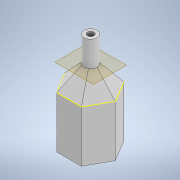
# Autodesk Inventor part: motorattacher
Saved by Autodesk Inventor 2022 (Build 260153000, 153)
## iProperties
Created: 2022-04-02
Part Number: motorattacher
Material: Generic
Document SubType Name: Modeling
Designer: moaze
Density: 1 g/cm^3
Appearance: Default
Author: moaze
Autodesk Inventor part; units mm, degrees
ref_plane "YZ Plane" through (0, 0, 0) normal (1, 0, 0) x (0, 1, 0)
ref_plane "XZ Plane" through (0, 0, 0) normal (0, 1, 0) x (-1, 0, 0)
ref_plane "XY Plane" through (0, 0, 0) normal (0, 0, 1) x (1, 0, 0)
sketch "Sketch1" plane through (0, 0, 0) normal (0, 1, 0) x (-1, 0, 0)
  line L0 (3.0315, -4.7903) -> (-2.5932, -4.7903)
  line L1 (-2.5932, -4.7903) -> (-5.3821, -0.0266)
  line L2 (-5.3821, -0.0266) -> (-2.721, 4.8097)
  line L3 (-2.721, 4.8097) -> (2.7981, 4.8097)
  line L4 (2.7981, 4.8097) -> (5.7396, 0.1397)
  line L5 (5.7396, 0.1397) -> (3.0315, -4.7903)
  line L6 (-7.5579, -0.0555) -> (-3.6782, -6.6826)
  line L7 (-3.6782, -6.6826) -> (4.1511, -6.6826)
  line L8 (4.1511, -6.6826) -> (7.9347, 0.2053)
  line L9 (7.9347, 0.2053) -> (3.8427, 6.7021)
  line L10 (3.8427, 6.7021) -> (-3.8397, 6.7021)
  line L11 (-3.8397, 6.7021) -> (-7.5579, -0.0555)
  line L12 (0.004, -1.2887) -> (0.004, -3.3542)
  dimension "d43" = 9.6
  constraints: 26 end point, 3 equal length, 2 perpendicular, 1 vertical, 5 other
  measures "d43" distance between parallel lines of L0 L3
ref_plane "Work Plane1" through (0, 14.35, 0) normal (0, 1, 0) x (1, 0, 0)
sketch "Sketch3" plane through (0, 14.35, 0) normal (0, 1, 0) x (1, 0, 0)
  circle A0 centre (0, 0) radius 2
  dimension "d7" = 4
  constraints: 1 centre point, 1 coincident
  measures "d7" diameter of A0
extrude "Extrusion3" add sketch "Sketch1" along normal blind 8
sketch "Sketch6" plane through (0, 8, 0) normal (0, 1, 0) x (1, 0, 0)
  line L0 (3.6782, 6.6826) -> (-4.1511, 6.6826) projected
  line L1 (-4.1511, 6.6826) -> (-7.9347, -0.2053) projected
  line L2 (-7.9347, -0.2053) -> (-3.8427, -6.7021) projected
  line L3 (-3.8427, -6.7021) -> (3.8397, -6.7021) projected
  line L4 (3.8397, -6.7021) -> (7.5579, 0.0555) projected
  line L5 (7.5579, 0.0555) -> (3.6782, 6.6826) projected
  line L6 (-3.0315, 4.7903) -> (2.5932, 4.7903) projected
  line L7 (2.5932, 4.7903) -> (5.3821, 0.0266) projected
  line L8 (5.3821, 0.0266) -> (2.721, -4.8097) projected
  line L9 (2.721, -4.8097) -> (-2.7981, -4.8097) projected
  line L10 (-2.7981, -4.8097) -> (-5.7396, -0.1397) projected
  line L11 (-5.7396, -0.1397) -> (-3.0315, 4.7903) projected
  point P0 (0, 0)
loft "Loft2" add profiles "Sketch3" section 1 edges at (-0.2365, 8, -6.6826) (-6.0429, 8, -3.2387) (-5.8887, 8, 3.4537) (-0.0015, 8, 6.7021) (5.6988, 8, 3.3233) (5.618, 8, -3.3691)
sketch "Sketch7" plane through (0, 14.35, 0) normal (0, 1, 0) x (0.9999645, 0, -0.0084267)
  arc A0 (1.0109, 1.7257) -> (-1.0109, 1.7257) centre (0, 0) ccw projected
  arc A1 (-1.0109, 1.7257) -> (-1.9997, -0.036) centre (0, 0) ccw projected
  arc A2 (-1.9997, -0.036) -> (-0.9777, -1.7447) centre (0, 0) ccw projected
  arc A3 (-0.9777, -1.7447) -> (1.0106, -1.7259) centre (0, 0) ccw projected
  arc A4 (1.0106, -1.7259) -> (2, -0.0025) centre (0, 0) ccw projected
  arc A5 (2, -0.0025) -> (1.0109, 1.7257) centre (0, 0) ccw projected
  point P0 (0, 0)
sketch "Sketch8" plane through (0, 0, 0) normal (0, -1, 0) x (1, 0, 0)
  line L0 (3.6782, -6.6826) -> (-4.1511, -6.6826) projected
  line L1 (7.5579, -0.0555) -> (3.6782, -6.6826) projected
  line L2 (3.8397, 6.7021) -> (7.5579, -0.0555) projected
  line L3 (-3.8427, 6.7021) -> (3.8397, 6.7021) projected
  line L4 (-7.9347, 0.2053) -> (-3.8427, 6.7021) projected
  line L5 (-4.1511, -6.6826) -> (-7.9347, 0.2053) projected
  line L6 (-3.0315, -4.7903) -> (2.5932, -4.7903) projected
  line L7 (-5.7396, 0.1397) -> (-3.0315, -4.7903) projected
  line L8 (-2.7981, 4.8097) -> (-5.7396, 0.1397) projected
  line L9 (2.721, 4.8097) -> (-2.7981, 4.8097) projected
  line L10 (5.3821, -0.0266) -> (2.721, 4.8097) projected
  line L11 (2.5932, -4.7903) -> (5.3821, -0.0266) projected
  point P0 (0, 0)
extrude "Extrusion4" add sketch "Sketch8" along normal blind 8
extrude "Extrusion5" add sketch "Sketch7" along normal blind 8
sketch "Sketch9" plane through (0, 22.35, 0) normal (0, 1, 0) x (1, 0, 0)
  point P0 (0, 0)
  point P1 (0, 0)
  constraints: 1 coincident
hole "Hole2" at (0, 22.35, 0) direction (0, -1, 0) diameter 2 end through all
body "Solid1"
